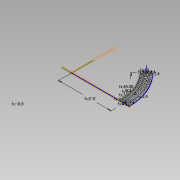
# Autodesk Inventor part: CurveRail-215-45
Saved by Autodesk Inventor 2021 (Build 250183000, 183)
## iProperties
Created: 2021-02-23
Part Number: CurveRail-215-45
Material: 一般
Document SubType Name: Modeling
Designer: kumagai
Density: 1 g/cm^3
Appearance: 既定
Author: kumagai
Autodesk Inventor part; units mm, degrees
ref_plane "XZ Plane" through (0, 0, 0) normal (0, 1, 0) x (-1, 0, 0)
sketch "outline" plane through (0, 0, 0) normal (0, 1, 0) x (-1, 0, 0)
  line L0 (0, -87.9029) -> (0, 24.4547) projected
  line L1 (-224.6399, 0) -> (37.44, 0) projected
  arc A0 (-234, 0) -> (-165.463, -165.463) centre (0, 0) ccw
  arc A1 (-196, 0) -> (-138.5929, -138.5929) centre (0, 0) ccw
  line L2 (0, 0) -> (-187.1999, 0)
  arc A2 (-221.5807, -11.9) -> (-158.5949, -155.2008) centre (0, 0) ccw
  arc A3 (-198, 0) -> (-140.0071, -140.0071) centre (0, 0) ccw
  arc A4 (-205.7, 0) -> (-145.4519, -145.4519) centre (0, 0) ccw
  arc A5 (-232, 0) -> (-164.0488, -164.0488) centre (0, 0) ccw
  arc A6 (-207.7595, -11.9) -> (-148.8362, -145.4421) centre (0, 0) ccw
  arc A7 (-224.3, 0) -> (-158.6041, -158.6041) centre (0, 0) ccw
  line L3 (-215, 8.4036) -> (-215, -7.4593)
  line L4 (-157.7637, -146.2922) -> (-125.244, -178.8119)
  line L5 (-155.3514, -155.3514) -> (-150.2602, -162.9881)
  line L6 (-150.2602, -162.9881) -> (-141.0678, -153.7957)
  line L7 (-141.0678, -153.7957) -> (-148.7046, -148.7046)
  line L8 (-154.9783, -151.5842) -> (-149.8872, -159.221)
  line L9 (-149.8872, -159.221) -> (-144.8349, -154.1687)
  line L10 (-144.8349, -154.1687) -> (-152.4717, -149.0776)
  line L11 (-138.5929, -138.5929) -> (-148.7046, -148.7046)
  line L12 (-155.3514, -155.3514) -> (-165.463, -165.463)
  line L13 (-148.8362, -145.4421) -> (-152.4717, -149.0776)
  line L14 (-154.9783, -151.5842) -> (-158.5949, -155.2008)
  line L15 (-207.7595, -11.9) -> (-221.5807, -11.9)
  line L16 (-210.2, 0) -> (-208.35, -9.5)
  line L17 (-208.35, -9.5) -> (-221.65, -9.5)
  line L18 (-221.65, -9.5) -> (-219.8, 0)
  line L19 (-196, 0) -> (-210.2, 0)
  line L20 (-219.8, 0) -> (-234, 0)
  point P0 (-234, 0)
  point P1 (-196, 0)
  dimension "d3" = 2
  dimension "d5" = 215
  dimension "d6" = 38
  dimension "d7" = 18.6
  dimension "d8" = 2.4
  dimension "d10" = 2.4
  dimension "d11" = 2.4
  dimension "d12" = 2.4
  dimension "d13" = 13
  dimension "d14" = 2.4
  dimension "d16" = 9.4
  dimension "d17" = 9
  dimension "d18" = 2.4
  dimension "d19" = 9.5
  dimension "d20" = 13.3
  dimension "d21" = 9.6
  dimension "d22" = 2.4
  dimension "d23" = 45
  constraints: 38 end point, 16 point on circle, 12 point on line, 8 centre point, 7 parallel, 6 coincident, 4 symmetric about line, 2 horizontal, 2 perpendicular, 1 vertical, 3 other
  measures "d3" radial gap between concentric circles of A1 A3
  measures "d5" distance between parallel lines of L3 L0
  measures "d6" radial gap between concentric circles of A0 A1
  measures "d7" radial gap between concentric circles of A4 A7
  measures "d8" radial gap between concentric circles of A4 A6
  measures "d10" distance between parallel lines of L9 L6
  measures "d11" distance between parallel lines of L5 L8
  measures "d12" distance between parallel lines of L7 L10
  measures "d13" distance of L5.end L6.end
  measures "d14" distance between parallel lines of L14 L12
  measures "d16" distance of L5.start L7.end
  measures "d17" distance between parallel lines of L11 L6
  measures "d18" radial gap between concentric circles of A7 A2
  measures "d19" distance between parallel lines of L19 L17
  measures "d20" distance of L17.end L16.end
  measures "d21" distance of L18.end L16.start
  measures "d22" distance between parallel lines of L17 L15
  measures "d23" angle of L19 L11
extrude "wall" add sketch "outline" along normal mid plane 8.4 contours L1 L18 L17 L16 A4 L11 L7 L6 L5 L12 A7 | A5 L12 A0 L20 | L1 A1 L11 A3
extrude "floor" add sketch "outline" along normal mid plane 2 contours L1 A7 L12 A5 L20 | L1 A3 L11 A4 | L15 A6 L13 L10 L9 L8 L14 A2
chamfer "C" distance 0.8 angle 45 24 edges at (182.9281, 1, -75.7713) (182.9281, -1, -75.7713) (190.042, 1, -78.718) (190.042, -1, -78.718) (207.2262, 1, -85.8359) (207.2262, -1, -85.8359) (214.3401, 1, -88.7826) (214.3401, -1, -88.7826) (203.1432, 1, -89.2887) (156.7866, 1, -153.3925) (152.4328, 1, -155.4026) (147.3611, 1, -156.6949) (148.6533, 1, -151.6232) (150.6539, 1, -147.2598) (190.3904, 1, -84.0067) (214.6701, 1, -11.9) (148.6533, -1, -151.6232) (147.3611, -1, -156.6949) (152.4328, -1, -155.4026) (156.7866, -1, -153.3925) (150.6539, -1, -147.2598) (203.1432, -1, -89.2887) (190.3904, -1, -84.0067) (214.6701, -1, -11.9)
sketch "スケッチ3" plane through (0, 1, 0) normal (0, 1, 0) x (1, 0, 0)
  line L0 (197.8, 0.025) -> (232.2, 0.025)
  line L1 (232.2, -0.025) -> (197.8, -0.025)
  line L2 (197.8, -0.025) -> (197.8, 0.025)
  line L3 (224.5, 0.025) -> (232.2, 0.025)
  line L4 (232.2, 0.025) -> (232.2, -0.025)
  line L5 (232.2, -0.025) -> (224.5, -0.025)
  line L6 (198, 0) -> (205.7, 0) projected
  line L7 (219.8, 0) -> (224.3, 0) projected
  line L8 (232, 0) -> (224.3, 0) projected
  line L9 (151.3014, 157.0997) -> (146.9563, 152.7545)
  line L10 (146.9563, 152.7545) -> (146.9987, 152.7262)
  line L11 (144.8349, 154.1687) -> (152.4717, 149.0776) projected
  line L12 (146.9987, 152.7262) -> (151.3297, 157.0572)
  line L13 (151.3297, 157.0572) -> (151.3014, 157.0997)
  line L14 (149.8872, 159.221) -> (154.9783, 151.5842) projected
  line L15 (144.8349, 154.1687) -> (149.8872, 159.221) projected
  point P0 (0, 0)
  dimension "d39" = 0.05
  dimension "d45" = 0.2
  dimension "d46" = 0.2
  dimension "d52" = 2.5
  dimension "d53" = 0.05
  constraints: 20 end point, 4 parallel, 4 point on line, 2 coincident, 2 horizontal, 1 perpendicular, 1 vertical, 2 other
  measures "d39" distance between parallel lines of L5 L3
  measures "d45" distance from line of L6.start L2
  measures "d46" distance from line of L4 L8.start
  measures "d52" distance between parallel lines of L9 L15
  measures "d53" distance between parallel lines of L12 L9
extrude "PrinterGuide" cut sketch "スケッチ3" against normal blind 0.2 contours L0 L4 L1 L2
pattern_circular "PrinterGuide_dist" count 56 over 45 about axis through (0, -10, 0) along (0, 1, 0) of "PrinterGuide"
sketch "スケッチ5" plane through (0, 4.2, 0) normal (0, 1, 0) x (1, 0, 0)
  line L0 (205.7, 0) -> (210.2, 0) projected
  line L1 (101.0338, 0) -> (210.2, 0)
  line L2 (210.2, 0) -> (208.35, 9.5) projected
  line L3 (210.2, 0) -> (208.35, 9.5)
  line L4 (208.35, 9.5) -> (221.65, 9.5)
  line L5 (221.65, 9.5) -> (219.8, 0) projected
  line L6 (221.65, 9.5) -> (219.8, 0)
  line L7 (219.8, 0) -> (221.0225, 0)
  line L8 (224.3, 0) -> (219.8, 0) projected
  line L9 (221.0225, 0) -> (223.1062, 10.7)
  line L10 (223.1062, 10.7) -> (206.8938, 10.7)
  line L11 (206.8938, 10.7) -> (208.9775, 0)
  point P0 (0, 0)
  dimension "d47" = 1.2
  dimension "d48" = 1.2
  dimension "d49" = 1.2
  constraints: 16 end point, 4 parallel, 3 collinear, 2 point on line
  measures "d47" distance between parallel lines of L9 L5
  measures "d48" distance between parallel lines of L10 L4
  measures "d49" distance between parallel lines of L2 L11
extrude "Cover" add sketch "スケッチ5" against normal through all
extrude "PrinterGuide2" cut sketch "スケッチ3" against normal blind 0.2 contours L13 L12 L10 L9
chamfer "面取り2" distance 0.5 angle 45 24 edges at (196, 0, 0) (198, 3, 0) (198, -3, 0) (205.7, 3, 0) (205.7, -3, 0) (210.2, 0, 0) (219.8, 0, 0) (224.3, 3, 0) (224.3, -3, 0) (232, 3, 0) (232, -3, 0) (234, 0, 0) (141.0678, 0, -153.7957) (150.2602, 0, -162.9881) (165.463, 0, -165.463) (164.0488, 3, -164.0488) (164.0488, -3, -164.0488) (158.6041, 3, -158.6041) (158.6041, -3, -158.6041) (145.4519, 3, -145.4519) (145.4519, -3, -145.4519) (140.0071, 3, -140.0071) (140.0071, -3, -140.0071) (138.5929, 0, -138.5929)
sketch "スケッチ6" plane through (198.8, -1, 0) normal (0, 0, 1) x (1, 0, 0)
  line L0 (-1.3, 5.2) -> (-1.3, 3.3) projected
  line L1 (7.4, 3.3) -> (7.4, 5.2) projected
  line L2 (25, 5.2) -> (25, 3.3) projected
  line L3 (33.7, 3.3) -> (33.7, 5.2) projected
  line L4 (-1.3, 5.2) -> (7.4, 5.2)
  line L5 (7.4, 5.2) -> (7.4, 4.7)
  line L6 (7.4, 4.7) -> (-1.3, 4.7)
  line L7 (-1.3, 4.7) -> (-1.3, 5.2)
  line L8 (25, 5.2) -> (33.7, 5.2)
  line L9 (33.7, 5.2) -> (33.7, 4.7)
  line L10 (33.7, 4.7) -> (25, 4.7)
  line L11 (25, 4.7) -> (25, 5.2)
  point P0 (-198.8, 1)
  dimension "d73" = 0.5
  constraints: 16 end point, 4 parallel, 3 point on line, 2 horizontal, 2 perpendicular
  measures "d73" distance between parallel lines of L10 L8
extrude "FillBlocker" add sketch "スケッチ6" along normal blind 0.3 and the other way blind 0.3
pattern_circular "円形状パターン2" count 2 over 45 about axis through (0, -10, 0) along (0, 1, 0) of "FillBlocker"
equation "\"d3\" = OuterWall"
equation "\"d5\" = CurveRadius"
equation "\"d6\" = RailWidth"
equation "\"d7\" = InsideWidth"
equation "\"d8\" = InnerWall"
equation "\"d10\" = InnerWall"
equation "\"d11\" = d10"
equation "\"d12\" = d10"
equation "\"d13\" = JointMW1 - 2 * cp"
equation "\"d14\" = d10"
equation "\"d16\" = JointMW2 - 2 * cp"
equation "\"d17\" = JointMH"
equation "\"d18\" = InnerWall"
equation "\"d19\" = JointFH"
equation "\"d20\" = JointFW1 + 2 * cp"
equation "\"d21\" = JointFW2 + 2 * cp"
equation "\"d22\" = InnerWall"
equation "\"d23\" = CurveAngle"
equation "\"d24\" = RailHeight"
equation "\"d26\" = RailHeight - 2 * RailDepth"
equation "\"d43\" = CurveAngle"
equation "\"CurveRadius\" = 215"
equation "\"CurveAngle\" = 45deg"
equation "\"d0\" = CurveAngle"
equation "\"d9\" = CurveAngle"
equation "\"OuterWall\" = 2"
equation "\"RailWidth\" = 38"
equation "\"InsideWidth\" = 18.6"
equation "\"InnerWall\" = 2.4"
equation "\"JointMW1\" = 13"
equation "\"cp\" = 0"
equation "\"JointMW2\" = 9.4"
equation "\"JointMH\" = 9"
equation "\"JointFH\" = 9.5"
equation "\"JointFW1\" = 13.3"
equation "\"JointFW2\" = 9.6"
equation "\"RailHeight\" = 8.4"
equation "\"RailDepth\" = 3.2"
